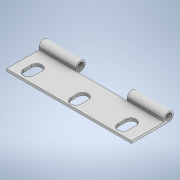
# Autodesk Inventor part: Ala 1 Bisagra tipo T
Saved by Autodesk Inventor 2020 (Build 240168000, 168)
## iProperties
Created: 2020-07-01
Part Number: Ala 1 Bisagra tipo T
Material: Genérico
Document SubType Name: Modeling
Designer: Pipi
Density: 1 g/cm^3
Appearance: Valor por defecto
Author: Pipi
Autodesk Inventor part; units mm, degrees
ref_plane "YZ Plane" through (0, 0, 0) normal (1, 0, 0) x (0, 1, 0)
ref_plane "XZ Plane" through (0, 0, 0) normal (0, 1, 0) x (-1, 0, 0)
ref_plane "XY Plane" through (0, 0, 0) normal (0, 0, 1) x (1, 0, 0)
sketch "Boceto1" plane through (0, 0, 0) normal (0, 1, 0) x (-1, 0, 0)
  line L0 (9.0866, 25.3081) -> (-54.4134, 25.3081)
  line L1 (-54.4134, 25.3081) -> (-54.4134, 8.8081)
  line L2 (-54.4134, 8.8081) -> (9.0866, 8.8081)
  line L3 (9.0866, 8.8081) -> (9.0866, 25.3081)
  arc A0 (-0.7134, 17.3081) -> (4.2866, 17.3081) centre (1.7866, 17.3081) ccw
  arc A1 (-25.1634, 18.3081) -> (-20.1634, 18.3081) centre (-22.6634, 18.3081) ccw
  arc A2 (-48.6134, 17.3081) -> (-43.6134, 17.3081) centre (-46.1134, 17.3081) ccw
  line L4 (4.2866, 17.3081) -> (4.2866, 21.3081)
  line L5 (-0.7134, 17.3081) -> (-0.7134, 21.3081)
  arc A3 (4.2866, 21.3081) -> (-0.7134, 21.3081) centre (1.7866, 21.3081) ccw
  line L6 (-43.6134, 17.3081) -> (-43.6134, 21.3081)
  line L7 (-48.6134, 17.3081) -> (-48.6134, 21.3081)
  arc A4 (-43.6134, 21.3081) -> (-48.6134, 21.3081) centre (-46.1134, 21.3081) ccw
  line L8 (-20.1634, 18.3081) -> (-20.1634, 21.8081)
  line L9 (-25.1634, 18.3081) -> (-25.1634, 21.8081)
  arc A5 (-20.1634, 21.8081) -> (-25.1634, 21.8081) centre (-22.6634, 21.8081) ccw
  point P0 (0, 0)
  dimension "d1" = 16.5
  dimension "d2" = 5
  dimension "d3" = 5
  dimension "d4" = 5
  dimension "d10" = 7
  dimension "d11" = 31.75
  dimension "d12" = 8
  dimension "d13" = 8.3
  dimension "d14" = 63.5
  dimension "d15" = 8
  dimension "d16" = 7.3
  dimension "d30" = 4
  dimension "d31" = 4
  dimension "d32" = 4
  dimension "d33" = 4
  dimension "d34" = 3.5
  dimension "d35" = 3.5
  constraints: 20 end point, 12 point on circle, 9 tangent, 6 centre point, 6 vertical, 3 perpendicular, 1 horizontal
  measures "d1" distance of L0.end L1.end
  measures "d2" diameter of A0
  measures "d3" diameter of A1
  measures "d4" diameter of A2
  measures "d10" distance from line of L0 A1.centre
  measures "d11" distance from line of L1 A1.centre
  measures "d12" distance from line of L0 A2.centre
  measures "d13" distance from line of L1 A2.centre
  measures "d14" distance of L0.start L0.end
  measures "d15" distance from line of L0 A0.centre
  measures "d16" distance from line of L3 A0.centre
  measures "d30" distance of L4.start L4.end
  measures "d31" distance of L5.start L5.end
  measures "d32" distance of L6.start L6.end
  measures "d33" distance of L7.start L7.end
  measures "d34" distance of L8.start L8.end
  measures "d35" distance of L9.start L9.end
extrude "Extrusión1" add sketch "Boceto1" along normal blind 1.2
sketch "Boceto2" plane through (54.4134, 0, 25.3081) normal (1, 0, 0) x (0, 0, -1)
  circle A0 centre (18.875, 2.375) radius 2.375
  circle A1 centre (18.875, 2.375) radius 1.625
  line L0 (16.5, 0) -> (16.5, 1.2) projected
  line L1 (0, 0) -> (16.5, 0) projected
  line L2 (16.5, 0) -> (16.5, 1.2) projected
  line L3 (16.5, 1.2) -> (16.5, 2.375)
  line L4 (16.5, 1.2) -> (16.5, 0)
  line L5 (16.5, 0) -> (18.875, 0)
  point P0 (25.3081, 0)
  dimension "d19" = 4.75
  dimension "d20" = 3.25
  constraints: 6 end point, 4 tangent, 2 centre point, 2 point on circle, 1 coincident, 1 collinear
  measures "d19" diameter of A0
  measures "d20" diameter of A1
extrude "Extrusión2" add sketch "Boceto2" against normal blind 63.5
sketch "Boceto3" plane through (0, 0, 0) normal (0, -1, 0) x (1, 0, 0)
  line L0 (54.4134, 8.8081) -> (-9.0866, 8.8081) projected
  line L1 (-9.0866, 8.8081) -> (54.4134, 8.8081)
  line L2 (22.6634, 8.8081) -> (35.6634, 8.8081)
  line L3 (35.6634, 8.8081) -> (9.6634, 8.8081)
  line L4 (9.6634, 8.8081) -> (9.6634, -4.6873)
  line L5 (9.6634, -4.6873) -> (35.6634, -4.6873)
  line L6 (35.6634, -4.6873) -> (35.6634, 8.8081)
  point P0 (0, 0)
  dimension "d23" = 13
  dimension "d24" = 26
  constraints: 12 end point, 3 perpendicular, 2 point on line, 1 collinear, 1 midpoint
  measures "d23" distance of L2.start L2.end
  measures "d24" distance of L2.end L3.end
extrude "Extrusión3" cut sketch "Boceto3" against normal blind 63.5
chamfer "Chaflán1" distance 0.25 angle 45 3 edges at (22.6634, 1.2, 15.8081) (-1.7866, 1.2, 14.8081) (46.1134, 1.2, 14.8081)
